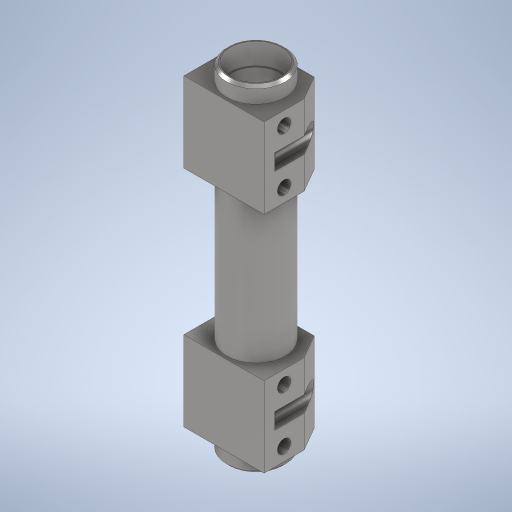
# Autodesk Inventor part: Wellengehäuse
Saved by Autodesk Inventor 2024 (Build 280153000, 153)
## iProperties
Created: 2024-03-15
Part Number: Wellengehäuse
Material: Stahl, galvanisiert
Document SubType Name: Modeling
Designer: ffogue
Density: 7.85 g/cm^3
Appearance: Galvanisiert
Author: ffogue
Autodesk Inventor part; units mm, degrees
sketch "Skizze1" plane through (0, 0, 0) normal (0, 0, 1) x (1, 0, 0)
  circle A0 centre (0, 0) radius 11
  dimension "d0" = 22
  constraints: 1 centre point, 1 coincident
  measures "d0" diameter of A0
extrude "Extrusion1" add sketch "Skizze1" against normal blind 126
ref_plane "Arbeitsebene1" through (0, 0, -6) normal (0, 0, 1) x (1, 0, 0)
sketch "Skizze2" plane through (0, 0, -6) normal (0, 0, 1) x (1, 0, 0)
  line L0 (-15, -12) -> (15, -12)
  line L1 (15, -12) -> (15, 12)
  line L2 (15, 12) -> (-15, 12)
  line L3 (-15, 12) -> (-15, -12)
  line L4 (-15, -12) -> (15, 12) construction
  line L5 (15, -12) -> (-15, 12) construction
  point P0 (0, 0)
  dimension "d4" = 24
  dimension "d5" = 30
  constraints: 12 end point, 2 midpoint, 2 parallel, 1 horizontal, 1 perpendicular
  measures "d4" distance between parallel lines of L0 L2
  measures "d5" distance between parallel lines of L1 L3
extrude "Extrusion2" add sketch "Skizze2" against normal blind 30
chamfer "Fasen1" distance 9 angle 30 1 edges at (15, 12, -21) measured on face at (15, -4, -16)
chamfer "Fasen2" distance 9 angle 30 1 edges at (-15, 12, -21) measured on face at (-15, 4, -16)
ref_plane "Arbeitsebene2" through (0, 0, -63) normal (0, 0, 1) x (1, 0, 0)
mirror "Spiegeln1" about plane through (0, 0, -63) normal (0, 0, 1) of "Extrusion2", "Fasen2", "Fasen1"
ref_plane "Arbeitsebene4" through (9.8038, 12, -120) normal (0, -1, 0) x (0, 0, -1)
sketch "Skizze4" plane through (9.8038, 12, -120) normal (0, -1, 0) x (0, 0, -1)
  line L0 (-30, 5.1962) -> (-30, 0) projected
  line L1 (0, 5.1962) -> (-30, 5.1962) projected
  line L2 (0, 0) -> (0, 5.1962) projected
  line L3 (-30, 0) -> (0, 0) projected
  line L4 (-18, 5.1962) -> (-18, 3.1962)
  arc A0 (-18, 3.1962) -> (-12, 3.1962) centre (-15, 3.1962) ccw
  line L5 (-12, 3.1962) -> (-12, 5.1962)
  point P0 (-120, -9.8038)
  point P1 (-15, 5.1962)
  dimension "d18" = 2
  dimension "d19" = 6
  constraints: 4 end point, 2 point on circle, 2 point on line, 2 tangent, 1 centre point, 1 midpoint, 1 perpendicular, 1 vertical, 1 vertical alignment
  measures "d18" distance from line of L1 A0.centre
  measures "d19" distance between parallel lines of L5 L4
extrude "Extrusion3" cut sketch "Skizze4" along normal blind 20 contours L1 L5 A0 L4
mirror "Spiegeln2" about plane through (0, 0, -63) normal (0, 0, 1) of "Extrusion3"
ref_plane "Arbeitsebene5" through (0, 0, 0) normal (1, 0, 0) x (0, 1, 0)
mirror "Spiegeln3" about plane through (0, 0, 0) normal (1, 0, 0) of "Extrusion3", "Spiegeln2"
sketch "Skizze5" plane through (13, -8, -18) normal (0, 1, 0) x (1, 0, 0)
  arc A0 (0, 6) -> (0, 0) centre (0, 3) ccw projected
  point P0 (-13, -18)
  constraints: 1 coincident
hole "Bohrung1" at (13, -8, -21) direction (0, -1, 0) diameter 2 depth 2
sketch "Skizze6" plane through (15, -12, -6) normal (1, 0, 0) x (0, 0, -1)
  line L0 (0, 0) -> (0, 15) projected
  line L1 (0, 0) -> (30, 0) projected
  line L2 (15, 0) -> (15, 23.6603) construction
  ellipse E0 centre (15, 18.4641) end of major axis (15, 23.6603) minor radius 3 (18, 18.4641) -> (12, 18.4641) ccw projected
  line L3 (114, 0) -> (84, 0) projected
  line L4 (99, 0) -> (99, 23.6603) construction
  ellipse E1 centre (99, 18.4641) end of major axis (99, 23.6603) minor radius 3 (102, 18.4641) -> (96, 18.4641) ccw projected
  line L5 (84, 15) -> (84, 0) projected
  point P0 (-6, 12)
  point P1 (5, 7.5)
  point P2 (0, 7.5)
  point P3 (25, 7.5)
  point P4 (89, 7.5)
  point P5 (109, 7.5)
  point P6 (84, 7.5)
  point P7 (84, 7.5)
  dimension "d30" = 5
  dimension "d31" = 5
  constraints: 5 midpoint, 4 end point, 4 horizontal alignment, 2 symmetric about line, 2 vertical, 4 other
  measures "d30" distance from line of point (5, 7.5) L0
  measures "d31" distance of point (89, 7.5) point (84, 7.5)
hole "Bohrung2" at (15, -4.5, -11) at (15, -4.5, -31) at (15, -4.5, -95) at (15, -4.5, -115) direction (-1, 0, 0) diameter 5 depth 30
sketch "Skizze7" plane through (0, 0, 0) normal (0, 0, 1) x (1, 0, 0)
  circle A0 centre (0, 0) radius 11 projected
  constraints: 1 coincident
hole "Bohrung3" at (0, 0, 0) direction (0, 0, -1) diameter 19 depth 8
sketch "Skizze8" plane through (0, 0, -8) normal (0, 0, 1) x (1, 0, 0)
  circle A0 centre (0, 0) radius 11 projected
  constraints: 1 coincident
hole "Bohrung4" at (0, 0, -8) direction (0, 0, -1) diameter 18 depth 118
chamfer "Fasen3" distance 1 angle 45 1 edges at (-11, 0, 0)
chamfer "Fasen4" distance 1 angle 45 1 edges at (-11, 0, -126)
